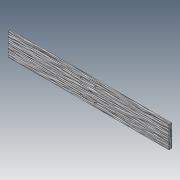
# Autodesk Inventor part: Bed bracket
Saved by Autodesk Inventor 2019 (Build 230136000, 136)
## iProperties
Created: 2018-11-26
Part Number: Bed bracket
Material: Fiberglass Batt
Document SubType Name: Modeling
Designer: LillaHunden
Density: 0.032 g/cm^3
Appearance: Gray
Mass: 105.389 g
Surface Area: 163.584 cm^2
Volume: 39.3244 cm^3
Author: LillaHunden
Autodesk Inventor part; units mm, degrees
ref_plane "YZ Plane" through (0, 0, 0) normal (1, 0, 0) x (0, 1, 0)
ref_plane "XZ Plane" through (0, 0, 0) normal (0, 1, 0) x (-1, 0, 0)
ref_plane "XY Plane" through (0, 0, 0) normal (0, 0, 1) x (1, 0, 0)
sketch "Sketch1" plane through (0, 0, 0) normal (1, 0, 0) x (0, 1, 0)
  line L0 (15, -2) -> (-15, -2)
  line L1 (-15, -2) -> (-15, 2)
  line L2 (-15, 2) -> (15, 2)
  line L3 (15, 2) -> (15, -2)
  line L4 (15, -2) -> (-15, 2) construction
  line L5 (-15, -2) -> (15, 2) construction
  point P0 (0, 0)
  dimension "d0" = 30
  dimension "d1" = 4
  constraints: 12 end point, 2 midpoint, 2 parallel, 1 horizontal, 1 perpendicular
  measures "d0" distance of L1.end L2.end
  measures "d1" distance of L0.end L1.end
extrude "Extrusion1" add sketch "Sketch1" along normal blind 220
sketch "Sketch2" plane through (0, -15, -2) normal (0, 0, -1) x (-1, 0, 0)
  point P0 (-100, 25)
  point P1 (-100, 5)
  point P2 (-120, 5)
  point P3 (-120, 25)
hole "Hole1" at (100, 10, -2) at (100, -10, -2) at (120, -10, -2) at (120, 10, -2) direction (0, 0, 1) diameter 3.4 depth 4 countersink diameter 6.3 countersink angle 90
body "Solid1"
